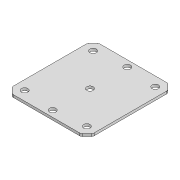
# Autodesk Inventor part: CCM_Mount_C
Saved by Autodesk Inventor 2020 (Build 240168000, 168)
## iProperties
Created: 2021-07-12
Part Number: CCM_Mount_C
Material: 一般
Document SubType Name: Modeling
Designer: magnarecta
Density: 1 g/cm^3
Appearance: 既定
Author: magnarecta
Autodesk Inventor part; units mm, degrees
ref_plane "YZ Plane" through (0, 0, 0) normal (1, 0, 0) x (0, 1, 0)
ref_plane "XZ Plane" through (0, 0, 0) normal (0, 1, 0) x (-1, 0, 0)
ref_plane "XY Plane" through (0, 0, 0) normal (0, 0, 1) x (1, 0, 0)
sketch "スケッチ1" plane through (0, 0, 0) normal (0, 1, 0) x (-1, 0, 0)
  line L0 (-32.5, -35) -> (32.5, -35)
  line L1 (32.5, -35) -> (32.5, 35)
  line L2 (32.5, 35) -> (-32.5, 35)
  line L3 (-32.5, 35) -> (-32.5, -35)
  line L4 (-32.5, -35) -> (32.5, 35) construction
  line L5 (32.5, -35) -> (-32.5, 35) construction
  point P0 (0, 0)
  dimension "d0" = 65
  dimension "d1" = 70
  constraints: 12 end point, 2 midpoint, 2 parallel, 1 horizontal, 1 perpendicular
  measures "d0" distance of L0.start L0.end
  measures "d1" distance of L0.end L1.end
extrude "押し出し1" add sketch "スケッチ1" along normal blind 2
sketch "スケッチ2" plane through (0, 2, 0) normal (0, 1, 0) x (1, 0, 0)
  line L0 (25, 27.5) -> (-25, 27.5)
  line L1 (-25, 27.5) -> (-25, -27.5)
  line L2 (-25, -27.5) -> (25, -27.5)
  line L3 (25, -27.5) -> (25, 27.5)
  line L4 (25, 27.5) -> (-25, -27.5) construction
  line L5 (-25, 27.5) -> (25, -27.5) construction
  point P0 (0, 0)
  dimension "d4" = 50
  dimension "d5" = 55
  constraints: 12 end point, 2 midpoint, 2 parallel, 1 horizontal, 1 perpendicular
  measures "d4" distance of L2.end L1.end
  measures "d5" distance of L1.end L0.end
hole "穴1" at (-25, 2, 27.5) at (25, 2, 27.5) at (25, 2, -27.5) at (-25, 2, -27.5) direction (0, -1, 0) diameter 5.2 depth 8 tip angle 118
chamfer "面取り1" distance 5 angle 45 4 edges at (-32.5, 1, 35) (32.5, 1, 35) (32.5, 1, -35) (-32.5, 1, -35)
fillet "フィレット3" radius 2 8 edges at (-27.5, 1, 35) (27.5, 1, 35) (32.5, 1, 30) (32.5, 1, -30) (27.5, 1, -35) (-32.5, 1, -30) (-27.5, 1, -35) (-32.5, 1, 30)
sketch "スケッチ5" plane through (0, 2, 0) normal (0, 1, 0) x (1, 0, 0)
  arc A0 (-32.5, -29.1716) -> (-31.9142, -30.5858) centre (-30.5, -29.1716) ccw projected
  line L0 (-28.0858, -34.4142) -> (-31.9142, -30.5858) projected
  arc A1 (-28.0858, -34.4142) -> (-26.6716, -35) centre (-26.6716, -33) ccw projected
  line L1 (-26.6716, -35) -> (26.6716, -35) projected
  arc A2 (26.6716, -35) -> (28.0858, -34.4142) centre (26.6716, -33) ccw projected
  line L2 (31.9142, -30.5858) -> (28.0858, -34.4142) projected
  arc A3 (31.9142, -30.5858) -> (32.5, -29.1716) centre (30.5, -29.1716) ccw projected
  line L3 (32.5, -29.1716) -> (32.5, 29.1716) projected
  arc A4 (32.5, 29.1716) -> (31.9142, 30.5858) centre (30.5, 29.1716) ccw projected
  line L4 (28.0858, 34.4142) -> (31.9142, 30.5858) projected
  arc A5 (28.0858, 34.4142) -> (26.6716, 35) centre (26.6716, 33) ccw projected
  line L5 (26.6716, 35) -> (-26.6716, 35) projected
  arc A6 (-26.6716, 35) -> (-28.0858, 34.4142) centre (-26.6716, 33) ccw projected
  line L6 (-31.9142, 30.5858) -> (-28.0858, 34.4142) projected
  arc A7 (-31.9142, 30.5858) -> (-32.5, 29.1716) centre (-30.5, 29.1716) ccw projected
  line L7 (-32.5, 29.1716) -> (-32.5, -29.1716) projected
  circle A8 centre (25, 27.5) radius 2.6 projected
  circle A9 centre (-25, -27.5) radius 2.6 projected
  circle A10 centre (25, -27.5) radius 2.6 projected
  circle A11 centre (-25, 27.5) radius 2.6 projected
  point P0 (0, 0)
  point P1 (0, 30)
  point P2 (0, -30)
  point P3 (0, 0)
  dimension "d32" = 5
  dimension "d33" = 5
  constraints: 1 coincident
  measures "d32" distance from line of point (0, -30) L1
  measures "d33" distance from line of L5 point (0, 30)
hole "穴3" at (0, 2, -30) at (0, 2, 30) at (0, 2, 0) direction (0, -1, 0) diameter 5.2 depth 11.8 tip angle 118
